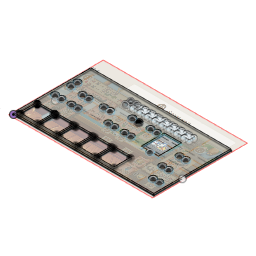
Maracaibo Overlay (Autodesk Fusion 360 design; units mm, degrees)
Autodesk Fusion 360 part; units mm, degrees
sketch "Sketch1" plane through (0, 0, 0) normal (0, 1, 0) x (1, 0, 0)
  line L0 (0, 0) -> (245, 0)
  line L1 (245, 0) -> (245, 135)
  line L2 (245, 135) -> (0, 135)
  line L3 (0, 135) -> (0, 0)
  line L4 (6, 36.5) -> (35, 36.5)
  line L5 (36, 35.5) -> (36, 6.5)
  line L6 (35, 5.5) -> (6, 5.5)
  line L7 (5, 6.5) -> (5, 35.5)
  circle A0 centre (19.8735, 63.7677) radius 5.5
  circle A1 centre (32.4098, 87.9753) radius 5.5
  circle A2 centre (43.4109, 87.9753) radius 5.5
  circle A3 centre (9.2367, 91.4502) radius 5.5
  circle A4 centre (9.2367, 102.5395) radius 5.5
  circle A5 centre (37.4037, 63.7677) radius 5.5
  circle A6 centre (48.4472, 63.7677) radius 5.5
  circle A7 centre (69.5756, 87.9753) radius 5.5
  circle A8 centre (80.5766, 87.9753) radius 5.5
  circle A9 centre (111.4393, 96) radius 5.5
  circle A10 centre (122.5, 96) radius 5.5
  circle A11 centre (97.9168, 67.5) radius 5.5
  circle A12 centre (108.962, 67.5) radius 5.5
  circle A13 centre (126.3779, 67.5) radius 5.5
  circle A14 centre (137.3818, 67.5) radius 5.5
  circle A15 centre (154.4171, 96) radius 5.5
  circle A16 centre (143.3532, 96) radius 5.5
  circle A17 centre (210, 79.9653) radius 5.5
  circle A18 centre (221.0157, 79.9653) radius 5.5
  circle A19 centre (8.83, 63.7677) radius 5.5
  circle A20 centre (210, 49.9285) radius 5.5
  circle A21 centre (221.0994, 49.9285) radius 5.5
  circle A22 centre (220.9449, 22.886) radius 5.5
  circle A23 centre (231.9924, 22.886) radius 5.5
  line L8 (83.668, 122.1819) -> (91.668, 122.1819)
  line L9 (92.668, 121.1819) -> (92.668, 113.1819)
  line L10 (91.668, 112.1819) -> (83.668, 112.1819)
  line L11 (82.668, 113.1819) -> (82.668, 121.1819)
  arc A24 (6, 36.5) -> (5, 35.5) centre (6, 35.5) ccw
  arc A25 (36, 35.5) -> (35, 36.5) centre (35, 35.5) ccw
  arc A26 (35, 5.5) -> (36, 6.5) centre (35, 6.5) ccw
  arc A27 (5, 6.5) -> (6, 5.5) centre (6, 6.5) ccw
  arc A28 (69.5, 35.5) -> (68.5, 36.5) centre (68.5, 35.5) ccw
  line L12 (69.5, 35.5) -> (69.5, 6.5)
  arc A29 (68.5, 5.5) -> (69.5, 6.5) centre (68.5, 6.5) ccw
  line L13 (68.5, 5.5) -> (39.5, 5.5)
  arc A30 (38.5, 6.5) -> (39.5, 5.5) centre (39.5, 6.5) ccw
  line L14 (38.5, 6.5) -> (38.5, 35.5)
  arc A31 (39.5, 36.5) -> (38.5, 35.5) centre (39.5, 35.5) ccw
  line L15 (39.5, 36.5) -> (68.5, 36.5)
  arc A32 (103, 35.5) -> (102, 36.5) centre (102, 35.5) ccw
  line L16 (103, 35.5) -> (103, 6.5)
  arc A33 (102, 5.5) -> (103, 6.5) centre (102, 6.5) ccw
  line L17 (102, 5.5) -> (73, 5.5)
  arc A34 (72, 6.5) -> (73, 5.5) centre (73, 6.5) ccw
  line L18 (72, 6.5) -> (72, 35.5)
  arc A35 (73, 36.5) -> (72, 35.5) centre (73, 35.5) ccw
  line L19 (73, 36.5) -> (102, 36.5)
  arc A36 (136.5, 35.5) -> (135.5, 36.5) centre (135.5, 35.5) ccw
  line L20 (136.5, 35.5) -> (136.5, 6.5)
  arc A37 (135.5, 5.5) -> (136.5, 6.5) centre (135.5, 6.5) ccw
  line L21 (135.5, 5.5) -> (106.5, 5.5)
  arc A38 (105.5, 6.5) -> (106.5, 5.5) centre (106.5, 6.5) ccw
  line L22 (105.5, 6.5) -> (105.5, 35.5)
  arc A39 (106.5, 36.5) -> (105.5, 35.5) centre (106.5, 35.5) ccw
  line L23 (106.5, 36.5) -> (135.5, 36.5)
  arc A40 (170, 35.5) -> (169, 36.5) centre (169, 35.5) ccw
  line L24 (170, 35.5) -> (170, 6.5)
  arc A41 (169, 5.5) -> (170, 6.5) centre (169, 6.5) ccw
  line L25 (169, 5.5) -> (140, 5.5)
  arc A42 (139, 6.5) -> (140, 5.5) centre (140, 6.5) ccw
  line L26 (139, 6.5) -> (139, 35.5)
  arc A43 (140, 36.5) -> (139, 35.5) centre (140, 35.5) ccw
  line L27 (140, 36.5) -> (169, 36.5)
  line L28 (0, 87.9753) -> (245, 87.9753) construction
  line L29 (0, 63.7677) -> (245, 63.7677) construction
  line L30 (0, 67.5) -> (245, 67.5) construction
  line L31 (0, 96) -> (245, 96) construction
  line L32 (210, 135) -> (210, 0) construction
  line L33 (210, 79.9653) -> (245, 79.9653) construction
  line L34 (210, 49.9285) -> (245, 49.9285) construction
  line L35 (220.9449, 22.886) -> (245, 22.886) construction
  arc A44 (83.668, 122.1819) -> (82.668, 121.1819) centre (83.668, 121.1819) ccw
  arc A45 (92.668, 121.1819) -> (91.668, 122.1819) centre (91.668, 121.1819) ccw
  arc A46 (91.668, 112.1819) -> (92.668, 113.1819) centre (91.668, 113.1819) ccw
  arc A47 (82.668, 113.1819) -> (83.668, 112.1819) centre (83.668, 113.1819) ccw
  arc A48 (105.418, 121.1819) -> (104.418, 122.1819) centre (104.418, 121.1819) ccw
  line L36 (105.418, 121.1819) -> (105.418, 113.1819)
  arc A49 (104.418, 112.1819) -> (105.418, 113.1819) centre (104.418, 113.1819) ccw
  line L37 (104.418, 112.1819) -> (96.418, 112.1819)
  arc A50 (95.418, 113.1819) -> (96.418, 112.1819) centre (96.418, 113.1819) ccw
  line L38 (95.418, 113.1819) -> (95.418, 121.1819)
  arc A51 (96.418, 122.1819) -> (95.418, 121.1819) centre (96.418, 121.1819) ccw
  line L39 (96.418, 122.1819) -> (104.418, 122.1819)
  arc A52 (118.168, 121.1819) -> (117.168, 122.1819) centre (117.168, 121.1819) ccw
  line L40 (118.168, 121.1819) -> (118.168, 113.1819)
  arc A53 (117.168, 112.1819) -> (118.168, 113.1819) centre (117.168, 113.1819) ccw
  line L41 (117.168, 112.1819) -> (109.168, 112.1819)
  arc A54 (108.168, 113.1819) -> (109.168, 112.1819) centre (109.168, 113.1819) ccw
  line L42 (108.168, 113.1819) -> (108.168, 121.1819)
  arc A55 (109.168, 122.1819) -> (108.168, 121.1819) centre (109.168, 121.1819) ccw
  line L43 (109.168, 122.1819) -> (117.168, 122.1819)
  arc A56 (130.918, 121.1819) -> (129.918, 122.1819) centre (129.918, 121.1819) ccw
  line L44 (130.918, 121.1819) -> (130.918, 113.1819)
  arc A57 (129.918, 112.1819) -> (130.918, 113.1819) centre (129.918, 113.1819) ccw
  line L45 (129.918, 112.1819) -> (121.918, 112.1819)
  arc A58 (120.918, 113.1819) -> (121.918, 112.1819) centre (121.918, 113.1819) ccw
  line L46 (120.918, 113.1819) -> (120.918, 121.1819)
  arc A59 (121.918, 122.1819) -> (120.918, 121.1819) centre (121.918, 121.1819) ccw
  line L47 (121.918, 122.1819) -> (129.918, 122.1819)
  arc A60 (143.668, 121.1819) -> (142.668, 122.1819) centre (142.668, 121.1819) ccw
  line L48 (143.668, 121.1819) -> (143.668, 113.1819)
  arc A61 (142.668, 112.1819) -> (143.668, 113.1819) centre (142.668, 113.1819) ccw
  line L49 (142.668, 112.1819) -> (134.668, 112.1819)
  arc A62 (133.668, 113.1819) -> (134.668, 112.1819) centre (134.668, 113.1819) ccw
  line L50 (133.668, 113.1819) -> (133.668, 121.1819)
  arc A63 (134.668, 122.1819) -> (133.668, 121.1819) centre (134.668, 121.1819) ccw
  line L51 (134.668, 122.1819) -> (142.668, 122.1819)
  arc A64 (156.418, 121.1819) -> (155.418, 122.1819) centre (155.418, 121.1819) ccw
  line L52 (156.418, 121.1819) -> (156.418, 113.1819)
  arc A65 (155.418, 112.1819) -> (156.418, 113.1819) centre (155.418, 113.1819) ccw
  line L53 (155.418, 112.1819) -> (147.418, 112.1819)
  arc A66 (146.418, 113.1819) -> (147.418, 112.1819) centre (147.418, 113.1819) ccw
  line L54 (146.418, 113.1819) -> (146.418, 121.1819)
  arc A67 (147.418, 122.1819) -> (146.418, 121.1819) centre (147.418, 121.1819) ccw
  line L55 (147.418, 122.1819) -> (155.418, 122.1819)
  arc A68 (169.168, 121.1819) -> (168.168, 122.1819) centre (168.168, 121.1819) ccw
  line L56 (169.168, 121.1819) -> (169.168, 113.1819)
  arc A69 (168.168, 112.1819) -> (169.168, 113.1819) centre (168.168, 113.1819) ccw
  line L57 (168.168, 112.1819) -> (160.168, 112.1819)
  arc A70 (159.168, 113.1819) -> (160.168, 112.1819) centre (160.168, 113.1819) ccw
  line L58 (159.168, 113.1819) -> (159.168, 121.1819)
  arc A71 (160.168, 122.1819) -> (159.168, 121.1819) centre (160.168, 121.1819) ccw
  line L59 (160.168, 122.1819) -> (168.168, 122.1819)
  arc A72 (181.918, 121.1819) -> (180.918, 122.1819) centre (180.918, 121.1819) ccw
  line L60 (181.918, 121.1819) -> (181.918, 113.1819)
  arc A73 (180.918, 112.1819) -> (181.918, 113.1819) centre (180.918, 113.1819) ccw
  line L61 (180.918, 112.1819) -> (172.918, 112.1819)
  arc A74 (171.918, 113.1819) -> (172.918, 112.1819) centre (172.918, 113.1819) ccw
  line L62 (171.918, 113.1819) -> (171.918, 121.1819)
  arc A75 (172.918, 122.1819) -> (171.918, 121.1819) centre (172.918, 121.1819) ccw
  line L63 (172.918, 122.1819) -> (180.918, 122.1819)
  arc A76 (194.668, 121.1819) -> (193.668, 122.1819) centre (193.668, 121.1819) ccw
  line L64 (194.668, 121.1819) -> (194.668, 113.1819)
  arc A77 (193.668, 112.1819) -> (194.668, 113.1819) centre (193.668, 113.1819) ccw
  line L65 (193.668, 112.1819) -> (185.668, 112.1819)
  arc A78 (184.668, 113.1819) -> (185.668, 112.1819) centre (185.668, 113.1819) ccw
  line L66 (184.668, 113.1819) -> (184.668, 121.1819)
  arc A79 (185.668, 122.1819) -> (184.668, 121.1819) centre (185.668, 121.1819) ccw
  line L67 (185.668, 122.1819) -> (193.668, 122.1819)
  line L68 (9.2367, 91.4502) -> (9.2367, 135) construction
  line L69 (162.51, 100.7844) -> (192.51, 100.7844)
  line L70 (192.51, 100.7844) -> (192.51, 60.7844)
  line L71 (192.51, 60.7844) -> (162.51, 60.7844)
  line L72 (162.51, 60.7844) -> (162.51, 100.7844)
  circle A80 centre (177.51, 60.7844) radius 5
  point P0 (5, 36.5)
  point P1 (36, 36.5)
  point P2 (5, 5.5)
  point P3 (15.5352, 57.4855)
  point P4 (82.668, 122.1819)
  point P5 (92.668, 122.1819)
  point P6 (82.668, 112.1819)
  dimension "d1" = 245
  dimension "d2" = 135
  dimension "d5" = 31
  dimension "d6" = 31
  dimension "d7" = 5
  dimension "d8" = 5.5
  dimension "d38" = 11
  dimension "d39" = 11
  dimension "d40" = 11
  dimension "d41" = 11
  dimension "d42" = 11
  dimension "d43" = 11
  dimension "d44" = 11
  dimension "d45" = 11
  dimension "d46" = 11
  dimension "d47" = 11
  dimension "d48" = 11
  dimension "d49" = 11
  dimension "d50" = 11
  dimension "d51" = 11
  dimension "d52" = 11
  dimension "d53" = 11
  dimension "d54" = 11
  dimension "d55" = 11
  dimension "d56" = 11
  dimension "d57" = 11
  dimension "d59" = 11
  dimension "d60" = 11
  dimension "d61" = 11
  dimension "d62" = 11
  dimension "d63" = 10
  dimension "d64" = 10
  dimension "d65" = 1
  dimension "d68" = 134
  dimension "d69" = 0
  dimension "d82" = 39
  dimension "d83" = 1
  dimension "d86" = 102
  dimension "d87" = 0
  dimension "d88" = 30
  dimension "d89" = 40
  dimension "d90" = 10
  constraint horizontal L0
  constraint vertical L1
  constraint horizontal L2
  constraint vertical L3
  constraint coincident L0.start L3.end
  constraint horizontal L4
  constraint vertical L5
  constraint horizontal L6
  constraint vertical L7
  constraint horizontal L8
  constraint vertical L9
  constraint horizontal L10
  constraint vertical L11
  constraint coincident P0 L7
  constraint coincident P0 L4
  constraint tangent L7 A24
  constraint tangent L4 A24
  constraint coincident P1 L4
  constraint coincident P1 L5
  constraint tangent L4 A25
  constraint tangent L5 A25
  constraint equal A24 A25
  constraint tangent L6 A26
  constraint tangent L5 A26
  constraint equal A24 A26
  constraint coincident P2 L6
  constraint coincident P2 L7
  constraint tangent L6 A27
  constraint tangent L7 A27
  constraint equal A24 A27
  constraint coincident L3 L28.start
  constraint coincident L1 L28.end
  constraint perpendicular L1 L28
  constraint coincident L3 L29.start
  constraint coincident L1 L29.end
  constraint perpendicular L1 L29
  constraint coincident A0.centre L29
  constraint coincident A19.centre L29
  constraint coincident A5.centre L29
  constraint coincident A6.centre L29
  constraint coincident A1.centre L28
  constraint coincident A2.centre L28
  constraint coincident A7.centre L28
  constraint coincident A8.centre L28
  constraint midpoint L3 L30.start
  constraint midpoint L1 L30.end
  constraint coincident A11.centre L30
  constraint coincident A12.centre L30
  constraint coincident A13.centre L30
  constraint coincident A14.centre L30
  constraint coincident L3 L31.start
  constraint coincident L1 L31.end
  constraint perpendicular L1 L31
  constraint coincident A9.centre L31
  constraint midpoint A10.centre L31
  constraint coincident A16.centre L31
  constraint coincident A15.centre L31
  constraint coincident L2 L32.start
  constraint coincident L0 L32.end
  constraint perpendicular L0 L32
  constraint coincident A17.centre L32
  constraint coincident A17.centre L33.start
  constraint coincident L1 L33.end
  constraint perpendicular L1 L33
  constraint coincident A20.centre L34.start
  constraint perpendicular L32 L34
  constraint coincident A21.centre L34
  constraint coincident A18.centre L33
  constraint coincident A22.centre L35.start
  constraint coincident L1 L35.end
  constraint perpendicular L1 L35
  constraint coincident A23.centre L35
  constraint coincident P4 L11
  constraint coincident P4 L8
  constraint tangent L11 A44
  constraint tangent L8 A44
  constraint coincident P5 L8
  constraint coincident P5 L9
  constraint tangent L8 A45
  constraint tangent L9 A45
  constraint equal A44 A45
  constraint tangent L9 A46
  constraint tangent L10 A46
  constraint equal A44 A46
  constraint coincident P6 L10
  constraint coincident P6 L11
  constraint tangent L10 A47
  constraint tangent L11 A47
  constraint equal A44 A47
  constraint coincident A3.centre L68.start
  constraint coincident L2 L68.end
  constraint perpendicular L2 L68
  constraint coincident A4.centre L68
  constraint horizontal L69
  constraint vertical L70
  constraint horizontal L71
  constraint vertical L72
  constraint midpoint L71 A80.centre
  measures "d1" distance of L0.start L0.end
  measures "d2" distance of L0.start L2.end
  measures "d5" distance of P0 P1
  measures "d6" distance of P0 P2
  measures "d7" distance of L3 L7
  measures "d8" distance of L0 L6
  measures "d38" diameter of A0
  measures "d39" diameter of A1
  measures "d40" diameter of A2
  measures "d41" diameter of A3
  measures "d42" diameter of A4
  measures "d43" diameter of A5
  measures "d44" diameter of A6
  measures "d45" diameter of A7
  measures "d46" diameter of A8
  measures "d47" diameter of A9
  measures "d48" diameter of A10
  measures "d49" diameter of A11
  measures "d50" diameter of A12
  measures "d51" diameter of A13
  measures "d52" diameter of A14
  measures "d53" diameter of A15
  measures "d54" diameter of A16
  measures "d55" diameter of A17
  measures "d56" diameter of A18
  measures "d57" diameter of A19
  measures "d59" diameter of A20
  measures "d60" diameter of A21
  measures "d61" diameter of A22
  measures "d62" diameter of A23
  measures "d63" distance of P4 P6
  measures "d64" distance of P4 P5
  measures "d65" radius of A24
  measures "d82" distance of L2 L31
  measures "d83" radius of A44
  measures "d88" distance of L69.start L69.end
  measures "d89" distance of L69.start L71.end
  measures "d90" diameter of A80
extrude "Extrude1" add sketch "Sketch1" along normal blind 3 contours L0 L1 L2 L3 | A48 L36 A49 L37 A50 L38 A51 L39 | A52 L40 A53 L41 A54 L42 A55 L43 | A56 L44 A57 L45 A58 L46 A59 L47 | A60 L48 A61 L49 A62 L50 A63 L51 | A64 L52 A65 L53 A66 L54 A67 L55 | A68 L56 A69 L57 A70 L58 A71 L59 | A72 L60 A73 L61 A74 L62 A75 L63 | A76 L64 A77 L65 A78 L66 A79 L67 | L69 L70 L71 L72 A80 | L71 A80 | L71 A80
extrude "Extrude2" cut sketch "Sketch1" along normal blind 3 contours L69 L70 L71 L72 A80 | L71 A80 | L71 A80
extrude "Extrude3" cut sketch "Sketch1" along normal blind 3 contours A48 L36 A49 L37 A50 L38 A51 L39 | A52 L40 A53 L41 A54 L42 A55 L43 | A56 L44 A57 L45 A58 L46 A59 L47 | A60 L48 A61 L49 A62 L50 A63 L51 | A64 L52 A65 L53 A66 L54 A67 L55 | A68 L56 A69 L57 A70 L58 A71 L59 | A72 L60 A73 L61 A74 L62 A75 L63 | A76 L64 A77 L65 A78 L66 A79 L67
equation "disc = 11 mm"
equation "reward = 31 mm"
equation "d5 = reward"
equation "d6 = reward"
equation "d38 = disc"
equation "d39 = disc"
equation "d40 = disc"
equation "d41 = disc"
equation "d42 = disc"
equation "d43 = disc"
equation "d44 = disc"
equation "d45 = disc"
equation "d46 = disc"
equation "d47 = disc"
equation "d48 = disc"
equation "d49 = disc"
equation "d50 = disc"
equation "d51 = disc"
equation "d52 = disc"
equation "d53 = disc"
equation "d54 = disc"
equation "d55 = disc"
equation "d56 = disc"
equation "d57 = disc"
equation "d59 = disc"
equation "d60 = disc"
equation "d61 = disc"
equation "d62 = disc"
